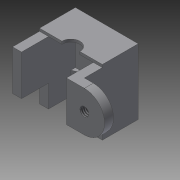
# Autodesk Inventor part: MotorMount
Saved by Autodesk Inventor 2013 (Build 170138000, 138)
## iProperties
Created: 2013-11-09
Part Number: MotorMount
Material: Generic
Document SubType Name: Modeling
Designer: JustinIndra
Density: 1 g/cm^3
Author: JustinIndra
Autodesk Inventor part; units mm, degrees
ref_plane "YZ Plane" through (0, 0, 0) normal (1, 0, 0) x (0, 1, 0)
ref_plane "XZ Plane" through (0, 0, 0) normal (0, 1, 0) x (-1, 0, 0)
ref_plane "XY Plane" through (0, 0, 0) normal (0, 0, 1) x (1, 0, 0)
sketch "Sketch1" plane through (0, 0, 0) normal (0, 0, 1) x (1, 0, 0)
  line L0 (-5, 6) -> (5, 6)
  line L1 (5, 6) -> (5, -6)
  line L2 (5, -6) -> (-5, -6)
  line L3 (-5, -6) -> (-5, 6)
  line L4 (-7, 8) -> (7, 8)
  line L5 (7, 8) -> (7, -6)
  line L6 (7, -6) -> (-7, -6)
  line L7 (-7, -6) -> (-7, 8)
  point P0 (0, 0)
  point P1 (0, 6)
  point P2 (-5, 0)
  point P3 (0, 8)
  dimension "d0" = 10
  dimension "d2" = 12
  dimension "d3" = 2
  dimension "d4" = 2
  constraints: 16 end point, 4 parallel, 3 midpoint, 2 horizontal, 2 perpendicular, 2 vertical alignment, 1 collinear, 1 horizontal alignment
  measures "d0" distance of L0.start L0.end
  measures "d2" distance of L2.end L0.start
  measures "d3" distance between parallel lines of L0 L4
  measures "d4" distance between parallel lines of L5 L1
extrude "Extrusion1" add sketch "Sketch1" along normal mid plane 9 contours L3 L6 L7 L4 L5 L1 L0
sketch "Sketch2" plane through (0, 0, 4.5) normal (0, 0, 1) x (1, 0, 0)
  line L0 (7, -6) -> (7, 8) projected
  line L1 (-7, 8) -> (7, 8)
  line L2 (7, 8) -> (7, 0)
  line L3 (7, 0) -> (-7, 0)
  line L4 (-7, 0) -> (-7, 8)
  point P0 (0, 0)
  point P1 (0, 0)
  constraints: 8 end point, 2 parallel, 1 coincident, 1 horizontal, 1 midpoint, 1 perpendicular, 1 point on line
extrude "Extrusion2" add sketch "Sketch2" along normal blind 0.6
sketch "Sketch3" plane through (0, 0, -4.5) normal (0, 0, -1) x (-1, 0, 0)
  line L0 (7, -6) -> (7, 8) projected
  line L1 (7, 8) -> (-7, 8) projected
  line L2 (-7, 8) -> (7, 8)
  line L3 (7, 8) -> (7, 0)
  line L4 (7, 0) -> (-7, 0)
  line L5 (-7, 0) -> (-7, 8)
  point P0 (0, 0)
  point P1 (0, 0)
  constraints: 8 end point, 2 parallel, 1 coincident, 1 horizontal, 1 midpoint, 1 perpendicular, 1 point on line
extrude "Extrusion3" add sketch "Sketch3" along normal blind 5
sketch "Sketch4" plane through (0, 0, -9.5) normal (0, 0, -1) x (-1, 0, 0)
  line L0 (-7, 0) -> (7, 0) projected
  line L1 (-5, 5) -> (5, 5)
  line L2 (5, 5) -> (5, 0)
  line L3 (5, 0) -> (-5, 0)
  line L4 (-5, 0) -> (-5, 5)
  line L5 (-5, -6) -> (-5, 0) projected
  line L6 (5, 0) -> (5, -6) projected
  arc A0 (5, 5) -> (-5, 5) centre (0, -5.9087) ccw
  line L7 (-5, 5) -> (5, 5)
  point P0 (0, 0)
  dimension "d11" = 5
  dimension "d14" = 12
  constraints: 10 end point, 3 collinear, 3 equal length, 2 point on circle, 1 centre point, 1 horizontal, 1 perpendicular
  measures "d11" distance of L1.end L2.end
  measures "d14" radius of A0
extrude "Extrusion4" cut sketch "Sketch4" against normal blind 5
sketch "Sketch5" plane through (0, 0, 5.1) normal (0, 0, 1) x (1, 0, 0)
  circle A0 centre (0, 0) radius 2
  dimension "d17" = 4
  constraints: 1 centre point, 1 coincident
  measures "d17" diameter of A0
extrude "Extrusion5" cut sketch "Sketch5" against normal through all
sketch "Sketch6" plane through (7, -6, 4.5) normal (1, 0, 0) x (0, 0, -1)
  line L0 (9, 6) -> (9, 0) projected
  line L1 (0, 0) -> (9, 0)
  line L2 (9, 0) -> (9, 2)
  line L3 (9, 2) -> (0, 2)
  line L4 (0, 2) -> (0, 0)
  point P0 (4.5, 6)
  dimension "d20" = 2
  constraints: 8 end point, 2 parallel, 1 horizontal, 1 perpendicular, 1 point on line
  measures "d20" distance between parallel lines of L1 L3
extrude "Extrusion6" add sketch "Sketch6" along normal blind 6.5
fillet "Fillet1" radius 4.5 2 edges at (13.5, -5, 4.5) (13.5, -5, -4.5)
sketch "Sketch8" plane through (7, -4, 4.5) normal (0, 1, 0) x (1, 0, 0)
  arc A0 (2, 0) -> (2, 9) centre (2, 4.5) ccw projected
  point P0 (-7, 4.5)
  constraints: 1 coincident
hole "Hole2" at (9, -4, 0) direction (0, -1, 0) diameter 2.013 end through all thread size "M2.5x0.45" class "6H" standard "ISO Metric profile"
equation "\"d4\" = d3"
body "Solid1"
